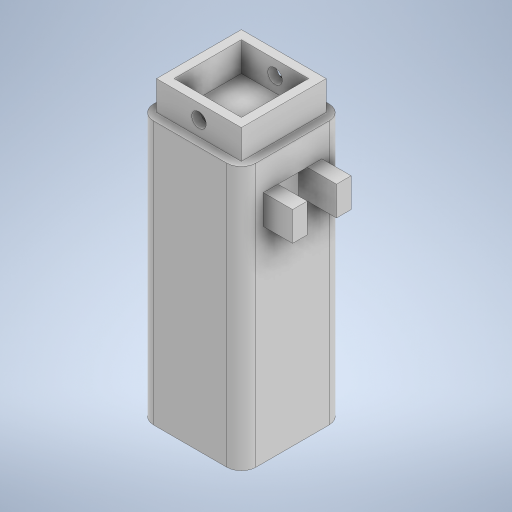
# Autodesk Inventor part: manico
Saved by Autodesk Inventor 2023 (Build 270158000, 158)
## iProperties
Created: 2023-08-01
Part Number: manico
Material: Generico
Document SubType Name: Modeling
Designer: Admin
Density: 1 g/cm^3
Appearance: Default
Author: Admin
Autodesk Inventor part; units mm, degrees
ref_plane "YZ Plane" through (0, 0, 0) normal (1, 0, 0) x (0, 1, 0)
ref_plane "XZ Plane" through (0, 0, 0) normal (0, 1, 0) x (-1, 0, 0)
ref_plane "XY Plane" through (0, 0, 0) normal (0, 0, 1) x (1, 0, 0)
sketch "Schizzo2" plane through (0, 0, 0) normal (0, 1, 0) x (-1, 0, 0)
  line L0 (11.5, 11.5) -> (-11.5, 11.5)
  line L1 (-11.5, 11.5) -> (-11.5, -11.5)
  line L2 (-11.5, -11.5) -> (11.5, -11.5)
  line L3 (11.5, -11.5) -> (11.5, 11.5)
  line L4 (17.5, 17.5) -> (-17.5, 17.5)
  line L5 (-17.5, 17.5) -> (-17.5, -17.5)
  line L6 (-17.5, -17.5) -> (17.5, -17.5)
  line L7 (17.5, -17.5) -> (17.5, 17.5)
  line L8 (0, 0) -> (13.1636, 0) construction
  line L9 (0, 0) -> (0, -15.8245) construction
  line L10 (14.5, 14.5) -> (-14.5, 14.5)
  line L11 (-14.5, 14.5) -> (-14.5, -14.5)
  line L12 (-14.5, -14.5) -> (14.5, -14.5)
  line L13 (14.5, -14.5) -> (14.5, 14.5)
  dimension "d1" = 23
  dimension "d2" = 35
  dimension "d3" = 3
  constraints: 28 end point, 6 parallel, 5 perpendicular, 3 horizontal, 1 vertical, 7 other
  measures "d1" distance of L1.end L2.end
  measures "d2" distance of L5.end L6.end
  measures "d3" distance between parallel lines of L3 L13
extrude "Estrusione1" add sketch "Schizzo2" along normal blind 10 and the other way blind 5 contours L13 L12 L11 L10
extrude "Estrusione2" add sketch "Schizzo2" against normal blind 90 contours L7 L6 L5 L4
extrude "Estrusione3" add sketch "Schizzo2" against normal blind 5 contours L3 L2 L1 L0
fillet "Raccordo1" radius 5 4 edges at (17.5, -45, 17.5) (17.5, -45, -17.5) (-17.5, -45, 17.5) (-17.5, -45, -17.5)
sketch "Schizzo3" plane through (0, 0, 0) normal (0, 0, 1) x (1, 0, 0)
  line L0 (-14.5, -5) -> (-14.5, 10) projected
  line L1 (-12.5, 0) -> (12.5, 0) projected
  line L2 (14.5, 10) -> (14.5, -5) projected
  line L3 (-14.5, 10) -> (14.5, 10) projected
  line L4 (0, 0) -> (0, 15.5409) construction
  line L5 (0, 0) -> (22.1267, 0) construction
  circle A0 centre (0, 5) radius 2.5
  dimension "d11" = 5
  dimension "d12" = 5
  constraints: 4 end point, 1 centre point, 1 horizontal, 1 point on line, 1 vertical
  measures "d11" diameter of A0
  measures "d12" distance from line of A0.centre L1
extrude "Estrusione4" cut sketch "Schizzo3" along normal through all both and the other way through all
sketch "Schizzo4" plane through (0, 0, 0) normal (1, 0, 0) x (0, 1, 0)
  line L0 (0, 12.5) -> (0, -12.5) projected
  line L1 (-90, -17.5) -> (0, -17.5) projected
  line L2 (0, 17.5) -> (-90, 17.5) projected
  line L3 (-90, -12.5) -> (-90, 12.5) projected
  line L4 (0, 0) -> (-112.8212, 0) construction
  line L5 (0, 0) -> (0, -73.2961) construction
  line L6 (-10, 10) -> (-20, 10)
  line L7 (-20, 10) -> (-20, -10)
  line L8 (-20, -10) -> (-10, -10)
  line L9 (-10, -10) -> (-10, 10)
  line L10 (-10, 5) -> (-20, 5)
  line L11 (-20, 5) -> (-20, -5)
  line L12 (-20, -5) -> (-10, -5)
  line L13 (-10, -5) -> (-10, 5)
  dimension "d17" = 10
  dimension "d18" = 20
  dimension "d19" = 10
  dimension "d20" = 10
  constraints: 20 end point, 4 parallel, 3 horizontal, 2 perpendicular, 2 point on line, 1 vertical, 2 other
  measures "d17" distance between parallel lines of L9 L0
  measures "d18" distance of L8.end L6.start
  measures "d19" distance of L7.end L8.end
  measures "d20" distance between parallel lines of L12 L10
extrude "Estrusione5" cut sketch "Schizzo4" along normal through all contours L9 L12 L7 L10
extrude "Estrusione6" add sketch "Schizzo4" along normal blind 27.5 contours L9 L10 L7 L6 | L9 L8 L7 L12
extrude "Estrusione7" cut sketch "Schizzo4" along normal up to surface (14.5 mm away) contours L9 L10 L7 L6 | L9 L8 L7 L12
